Autodesk Inventor part; units mm, degrees
(part 3 of 3)
sketch "Sketch7" plane through (0, 0, -31.75) normal (0, 0, -1) x (-1, 0, 0)
  line L0 (10.16, -55.8164) -> (-10.16, -55.8164)
  line L1 (-10.16, -55.8164) -> (-10.16, -62.1664)
  line L2 (-10.16, -62.1664) -> (10.16, -62.1664)
  line L3 (10.16, -62.1664) -> (10.16, -55.8164)
  line L4 (12.7, -54.4829) -> (12.7, -63.5) construction
  line L5 (12.7, -58.9914) -> (-12.7, -58.9914) construction
  line L6 (-12.7, -63.5) -> (-12.7, -54.4829) construction
  line L7 (12.7, -63.5) -> (-12.7, -63.5) construction
  line L8 (0, -63.5) -> (0, -58.9914) construction
  point P0 (0, 0)
  dimension "d22" = 6.35
  dimension "d23" = 20.32
  constraints: 12 end point, 4 midpoint, 2 parallel, 1 horizontal, 1 perpendicular, 2 other
  measures "d22" distance of L2.end L0.start
  measures "d23" distance of L0.start L0.end
extrude "Extrusion7" cut sketch "Sketch7" against normal up to surface (6.35 mm away)
pattern_circular "Circular Pattern1" count 4 over 360 about axis through (0, 0, 0) along (0, 0, -1) of "Extrusion7", "Extrusion6", "Extrusion5"
body "Solid1"
